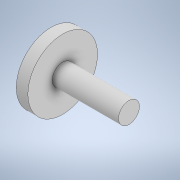
# Autodesk Inventor part: guia
Saved by Autodesk Inventor 2020 (Build 240168000, 168)
## iProperties
Created: 2021-03-26
Part Number: guia
Material: Generic
Document SubType Name: Modeling
Designer: super
Density: 1 g/cm^3
Appearance: Default
Author: super
Autodesk Inventor part; units mm, degrees
ref_plane "YZ Plane" through (0, 0, 0) normal (1, 0, 0) x (0, 1, 0)
ref_plane "XZ Plane" through (0, 0, 0) normal (0, 1, 0) x (-1, 0, 0)
ref_plane "XY Plane" through (0, 0, 0) normal (0, 0, 1) x (1, 0, 0)
sketch "Sketch1" plane through (0, 0, 0) normal (0, 0, 1) x (1, 0, 0)
  line L0 (8.367, 0) -> (8.367, 3)
  line L1 (8.367, 3) -> (-1.633, 3)
  line L2 (-1.633, 3) -> (-10.633, 3)
  line L3 (-10.633, 3) -> (-10.633, 9.9752)
  line L4 (-10.633, 9.9752) -> (-13.974, 9.9752)
  line L5 (-13.974, 9.9752) -> (-13.974, 0)
  line L6 (-13.974, 0) -> (8.367, 0)
  point P0 (0, 0)
  dimension "d0" = 3
  dimension "d1" = 10
  dimension "d3" = 9
  constraints: 14 end point, 5 perpendicular, 1 horizontal, 1 vertical
  measures "d0" distance of L0.start L0.end
  measures "d1" distance of L0.end L1.end
  measures "d3" distance of L1.end L2.end
revolve "Revolution1" add sketch "Sketch1" angle 360 about axis through (-13.974, 0, 0) along (1, 0, 0)
body "Solid1"
